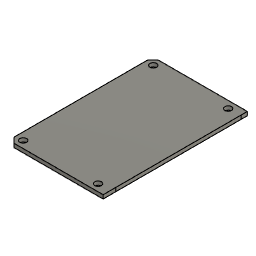
Side Panel - Blank Template (Autodesk Fusion 360 design; units mm, degrees)
Autodesk Fusion 360 part; units mm, degrees
sketch "sketch 2388" plane through (92, 0, 0) normal (1, 0, 0) x (0, 1, 0)
  circle A0 centre (-9.085, 9.5044) radius 1.8
  circle A1 centre (-79.085, 9.5044) radius 1.8
  circle A2 centre (-9.085, 49.8044) radius 1.8
  circle A3 centre (-79.085, 49.8044) radius 1.8
  line L0 (-8.1678, 53.8044) -> (-80.0022, 53.8044)
  line L1 (-80.0022, 53.8044) -> (-82.885, 50.9215)
  line L2 (-82.885, 50.9215) -> (-82.885, 3.0044)
  line L3 (-82.885, 3.0044) -> (-76.085, 3.0044)
  line L4 (-76.085, 3.0044) -> (-8.635, 3)
  line L5 (-8.635, 3) -> (-5.285, 3.0041)
  line L6 (-5.285, 3.0044) -> (-5.285, 3.0041)
  line L7 (-5.285, 50.9215) -> (-5.285, 3.0044)
  line L8 (-8.1678, 53.8044) -> (-5.285, 50.9215)
extrude "Extrude1" add sketch "sketch 2388" along normal blind -1.5 and the other way blind -0.5
move_body "Move1" bodies 1 to x (0, 0.000065, 1) y (-0.000065, 1, -0.000065) z (-1, -0.000065, 0) at (95.4994, -0.0058, -89.5006)
ref_plane "WorkPlane2" through (0, 0, 2.999) normal (0, 0, 1) x (1, 0, 0)
